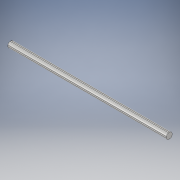
# Autodesk Inventor part: Axle
Saved by Autodesk Inventor 2018 (Build 220112000, 112)
## iProperties
Created: 2018-10-16
Part Number: Axle
Material: Generic
Document SubType Name: Modeling
Designer: 566609
Density: 1 g/cm^3
Appearance: Machined - Aluminum
Author: 566609
Autodesk Inventor part; units mm, degrees
ref_plane "YZ Plane" through (0, 0, 0) normal (1, 0, 0) x (0, 1, 0)
ref_plane "XZ Plane" through (0, 0, 0) normal (0, 1, 0) x (-1, 0, 0)
sketch "Sketch1" plane through (0, 0, 0) normal (1, 0, 0) x (0, 1, 0)
  line L0 (0, 0) -> (3, 0)
  line L1 (3, 0) -> (3, -3)
  line L2 (3, -3) -> (0, -3)
  line L3 (0, -3) -> (0, 0)
  dimension "d0" = 3
  dimension "d1" = 3
  constraints: 8 end point, 2 parallel, 1 horizontal, 1 perpendicular
  measures "d0" distance of L1.end L2.end
  measures "d1" distance of L0.end L1.end
extrude "Extrusion1" add sketch "Sketch1" along normal blind 85
fillet "Fillet1" radius 1.143 4 edges at (42.5, 3, 0) (42.5, 3, -3) (42.5, 0, 0) (42.5, 0, -3)
ref_plane "Work Plane1" through (0, 1.143, -1.5) normal (0, 0, 1) x (1, 0, 0)
body "Solid1"
